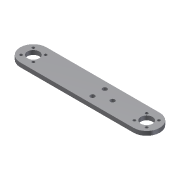
# Autodesk Inventor part: JointC4
Saved by Autodesk Inventor 2011 SP1 (Build 150282100, 282)
## iProperties
Created: 2012-10-23
Part Number: JointC4
Document SubType Name: Modeling
Designer: arihon
Density: 1 g/cm^3
Author: arihon
Autodesk Inventor part; units mm, degrees
ref_plane "YZ Plane" through (0, 0, 0) normal (1, 0, 0) x (0, 1, 0)
ref_plane "XZ Plane" through (0, 0, 0) normal (0, 1, 0) x (-1, 0, 0)
ref_plane "XY Plane" through (0, 0, 0) normal (0, 0, 1) x (1, 0, 0)
sketch "スケッチ1" plane through (0, 0, 0) normal (0, 0, 1) x (1, 0, 0)
  line L0 (-25, 9.4) -> (25, 9.4)
  line L1 (25, 9.4) -> (25, -9.4)
  line L2 (25, -9.4) -> (-25, -9.4)
  line L3 (-25, -9.4) -> (-25, 9.4)
  line L4 (25, 0) -> (-25, 0)
  circle A0 centre (11.2, 4.4) radius 1
  circle A1 centre (20, 4.4) radius 1
  circle A2 centre (11.2, -4.4) radius 1
  circle A3 centre (20, -4.4) radius 1
  point P0 (0, 0)
  dimension "d0" = 50
  dimension "d1" = 18.8
  dimension "d2" = 9.4
  dimension "d3" = 25
  dimension "d4" = 8.8
  dimension "d5" = 8.8
  dimension "d6" = 8.8
  dimension "d7" = 8.8
  dimension "d8" = 8.8
  dimension "d9" = 5
  dimension "d10" = 2
  dimension "d11" = 2
  dimension "d12" = 2
  dimension "d13" = 2
  constraints: 10 end point, 4 centre point, 4 coincident, 2 midpoint, 2 parallel, 1 horizontal, 1 perpendicular
  measures "d0" distance of L1.end L2.end
  measures "d1" distance of L2.end L0.start
  measures "d2" distance from line of L2 point (0, 0)
  measures "d3" distance from line of L3 point (0, 0)
  measures "d4" distance of point (11.2, 4.4) point (20, 4.4)
  measures "d5" distance of point (11.2, -4.4) point (20, -4.4)
  measures "d6" distance of point (20, -4.4) point (20, 4.4)
  measures "d7" distance of point (11.2, -4.4) point (11.2, 4.4)
  measures "d8" diameter of point (20, -4.4) L4
  measures "d9" distance from line of L1 point (20, -4.4)
  measures "d10" diameter of A0
  measures "d11" diameter of A1
  measures "d12" diameter of A2
  measures "d13" diameter of A3
extrude "押し出し1" add sketch "スケッチ1" along normal blind 3
fillet "フィレット1" radius 9.4 2 edges at (25, 9.4, 1.5) (25, -9.4, 1.5)
sketch "スケッチ2" plane through (0, 0, 3) normal (0, 0, 1) x (1, 0, 0)
  arc A0 (15.6, -9.4) -> (15.6, 9.4) centre (15.6, 0) ccw projected
  circle A1 centre (15.6, 0) radius 4.25
  point P0 (0, 0)
  dimension "d17" = 8.5
  constraints: 1 centre point, 1 coincident
  measures "d17" diameter of A1
extrude "押し出し2" cut sketch "スケッチ2" against normal through all
mirror "ミラー1" about plane through (-25, -9.4, 0) normal (-1, 0, 0)
sketch "スケッチ3" plane through (0, 0, 3) normal (0, 0, 1) x (1, 0, 0)
  arc A0 (15.6, -9.4) -> (15.6, 9.4) centre (15.6, 0) ccw projected
  line L0 (-65.6, 9.4) -> (15.6, 9.4) projected
  arc A1 (-65.6, 9.4) -> (-65.6, -9.4) centre (-65.6, 0) ccw projected
  line L1 (-65.6, 0) -> (15.6, 0)
  circle A2 centre (11.2, -4.4) radius 1 projected
  point P0 (0, 0)
  point P1 (-18.8, 4.4)
  point P2 (-18.8, -4.4)
  point P3 (-8.8, 0)
  dimension "d20" = 8.8
  dimension "d32" = 20
  dimension "d33" = 4.4
  dimension "d34" = 10
  dimension "d35" = 10
  constraints: 2 end point, 1 parallel, 1 point on line
  measures "d20" distance of point (-18.8, -4.4) point (-18.8, 4.4)
  measures "d32" horizontal distance of A2.centre point (-8.8, 0)
  measures "d33" distance from line of L1 point (-18.8, -4.4)
  measures "d34" horizontal distance of point (-18.8, 4.4) point (-8.8, 0)
  measures "d35" horizontal distance of point (-18.8, -4.4) point (-8.8, 0)
hole "Hole1" at (-18.8, 4.4, 3) at (-18.8, -4.4, 3) at (-8.8, 0, 3) direction (0, 0, -1) diameter 3.2 depth 8 tip angle 118
equation "\"d2\" = 0.5 * d1"
equation "\"d3\" = 0.5 * d0"
equation "\"d5\" = d4"
equation "\"d6\" = d4"
equation "\"d7\" = d4"
equation "\"d8\" = d4"
equation "\"d33\" = 0.5 * d20"
